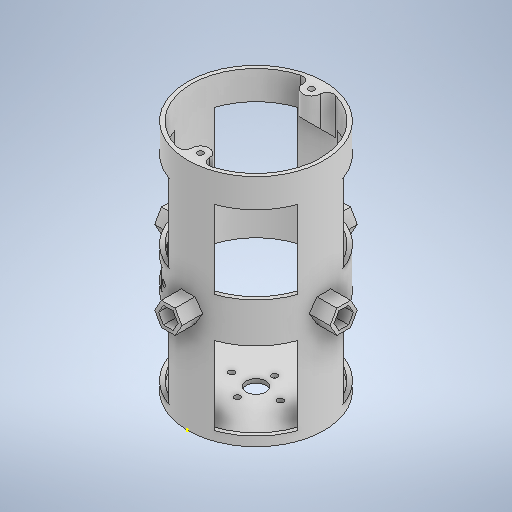
# Autodesk Inventor part: main_body
Saved by Autodesk Inventor 2025.3 (Build 293356000, 356)
## iProperties
Created: 2025-04-16
Part Number: main_body
Material: Generic
Document SubType Name: Modeling
Designer: Owner
Density: 1 g/cm^3
Appearance: Default
Author: Owner
Autodesk Inventor part; units mm, degrees
ref_plane "XZ Plane" through (0, 0, 0) normal (0, 1, 0) x (-1, 0, 0)
sketch "Sketch1" plane through (0, 0, 0) normal (0, 1, 0) x (-1, 0, 0)
  circle A0 centre (0, 0) radius 35
  dimension "d0" = 70
  constraints: 1 centre point, 1 coincident
  measures "d0" diameter of A0
extrude "Extrusion1" add sketch "Sketch1" along normal blind 120
shell "Shell1" thickness 2 removed faces 1 at (1.9985, 120, 11.019)
sketch "Sketch4" plane through (0, 120, 0) normal (0, 1, 0) x (1, 0, 0)
  circle A0 centre (0, 28.5) radius 4.5
  circle A1 centre (0, 0) radius 33 projected
  circle A2 centre (0, 28.5) radius 1.5
  line L0 (4.5, 28.5) -> (4.5, 32.6917)
  line L1 (0, 49) -> (0, -49) projected
  line L2 (-4.5, 28.5) -> (-4.5, 32.6917)
  point P0 (0, 33)
  dimension "d15" = 9
  dimension "d16" = 3
  constraints: 4 end point, 4 point on circle, 2 centre point, 2 tangent, 2 vertical, 1 coincident, 1 point on line
  measures "d15" diameter of A0
  measures "d16" diameter of A2
extrude "Extrusion2" add sketch "Sketch4" against normal blind 20 separate body contours A0 L1 A2 | A0 A1 L0 | L1 A2 A0 | A0 L2 A1
sketch "Sketch5" plane through (0, 0, 0) normal (1, 0, 0) x (0, 1, 0)
  line L0 (2, -33) -> (120, -33) projected
  line L1 (109, -24) -> (100, -33)
  line L2 (100, -24) -> (100, -28.5) projected
  line L3 (100, -33) -> (100, -24)
  line L4 (100, -24) -> (109, -24)
  point P0 (0, 0)
  point P1 (105.4104, -33)
  point P2 (130, -33)
  dimension "d60" = 45
  constraints: 6 end point, 3 point on line, 1 perpendicular, 1 vertical
  measures "d60" angle of L3 L1
extrude "Extrusion3" cut sketch "Sketch5" along normal mid plane 10 bodies 2
mirror "Mirror2" about plane through (0, 0, 0) normal (0, 0, 1) of "Extrusion3", "Extrusion2" bodies 2
combine bodies "Combine2" operation type add bodies to combine 2 1
sketch "Sketch6" plane through (0, 0, 0) normal (0, -1, 0) x (1, 0, 0)
  circle A0 centre (0, 9.5) radius 1.55
  circle A1 centre (0, -9.5) radius 1.55
  circle A2 centre (-12.5, 0) radius 1.55
  circle A3 centre (12.5, 0) radius 1.55
  circle A4 centre (0, 0) radius 20
  line L0 (0, 0) -> (14.1421, -14.1421)
  line L1 (0, -49) -> (0, 49) projected
  circle A5 centre (14.1421, -14.1421) radius 5
  circle A6 centre (0, 0) radius 5
  dimension "d69" = 40
  dimension "d35" = 3.1
  dimension "d36" = 3.1
  dimension "d37" = 3.1
  dimension "d38" = 3.1
  dimension "d39" = 19
  dimension "d40" = 25
  dimension "d41" = 9.5
  dimension "d42" = 12.5
  dimension "d71" = 45
  dimension "d72" = 10
  dimension "d73" = 10
  constraints: 6 centre point, 3 coincident, 2 end point, 3 other
  measures "d35" diameter of A0
  measures "d36" diameter of A1
  measures "d37" diameter of A2
  measures "d38" diameter of A3
  measures "d39" distance of A0.centre A1.centre
  measures "d40" distance of A2.centre A3.centre
  measures "d41" distance of point (0, 0) A0.centre
  measures "d42" distance of A3.centre point (0, 0)
  measures "d71" angle of L1 L0
  measures "d72" diameter of A5
  measures "d73" diameter of A6
extrude "Extrusion4" cut sketch "Sketch6" against normal through all contours A0 L1 | L1 A0 | A6 L0 L1 | L1 A6 | L0 A6 L1 | A5 A4 | A4 L0 A5 | A5 L0 A4 | L1 A1 | A1 L1 | A2 | A3 bodies 2
ref_plane "Work Plane1" through (0, 0, 35) normal (0, 0, 1) x (1, 0, 0)
sketch "Sketch7" plane through (0, 0, 35) normal (0, 0, 1) x (1, 0, 0)
  point P0 (0, 0)
sketch "Sketch8" plane through (0, 0, 35) normal (0, 0, 1) x (1, 0, 0)
  line L0 (2.5, 59.3301) -> (5, 55)
  line L1 (5, 55) -> (2.5, 50.6699)
  line L2 (2.5, 50.6699) -> (-2.5, 50.6699)
  line L3 (-2.5, 50.6699) -> (-5, 55)
  line L4 (-5, 55) -> (-2.5, 59.3301)
  line L5 (-2.5, 59.3301) -> (2.5, 59.3301)
  line L6 (35, 0) -> (-35, 0) projected
  line L7 (7, 55) -> (3.5, 48.9378)
  line L8 (3.5, 48.9378) -> (-3.5, 48.9378)
  line L9 (-3.5, 48.9378) -> (-7, 55)
  line L10 (-7, 55) -> (-3.5, 61.0622)
  line L11 (-3.5, 61.0622) -> (3.5, 61.0622)
  line L12 (3.5, 61.0622) -> (7, 55)
  point P0 (0, 0)
  point P1 (0, 55)
  point P2 (0, 55)
  point P3 (0, 48.9378)
  point P4 (0, 61.0622)
  dimension "d46" = 55
  dimension "d65" = 10
  dimension "d66" = 14
  constraints: 24 end point, 2 midpoint, 2 parallel, 1 coincident, 26 other
  measures "d46" distance from line of L6 point (0, 55)
  measures "d65" distance of L3.end L0.end
  measures "d66" distance of L9.end L7.start
extrude "Extrusion5" add sketch "Sketch8" against normal up to surface round surface about axis through (0, 0, 0) along (0, 1, 0) radius 35 far side no bodies 2
ref_plane "Work Plane2" through (0, 0, 0) normal (-0.7071068, 0, 0.7071068) x (0, -1, 0)
ref_plane "Work Plane3" through (-24.7487, 0, 24.7487) normal (-0.7071068, 0, 0.7071068) x (0, -1, 0)
sketch "Sketch10" plane through (-24.7487, 0, 24.7487) normal (-0.7071068, 0, 0.7071068) x (0, -1, 0)
  line L0 (-49.5, 7.75) -> (-60.5, 7.75)
  line L1 (-60.5, 7.75) -> (-60.5, -7.75)
  line L2 (-60.5, -7.75) -> (-49.5, -7.75)
  line L3 (-49.5, -7.75) -> (-49.5, 7.75)
  line L4 (-49.5, 7.75) -> (-60.5, -7.75) construction
  line L5 (-60.5, 7.75) -> (-49.5, -7.75) construction
  circle A0 centre (-55, -10.25) radius 2.5
  circle A1 centre (-55, -10.25) radius 1.5
  line L6 (12.1, 0) -> (-72.6, 0) projected
  circle A2 centre (-55, 10.25) radius 2.5
  circle A3 centre (-55, 10.25) radius 1.5
  line L7 (0, 35) -> (0, -35) projected
  point P0 (0, 0)
  point P1 (-55, 0)
  dimension "d54" = 11
  dimension "d55" = 15.5
  dimension "d56" = 5
  dimension "d57" = 3
  dimension "d67" = 55
  dimension "d68" = 55
  constraints: 12 end point, 4 centre point, 2 coincident, 2 midpoint, 2 parallel, 2 symmetric about line, 1 horizontal, 1 perpendicular, 1 point on line, 1 tangent, 2 other
  measures "d54" distance of L2.end L1.end
  measures "d55" distance of L1.end L0.end
  measures "d56" diameter of A0
  measures "d57" diameter of A1
  measures "d67" distance of point (0, 0) point (-55, 0)
  measures "d68" distance from line of L7 A0.centre
extrude "Extrusion7" cut sketch "Sketch10" against normal up to surface contours L3 L6 L1 L0 | L3 L2 L1 L6 | A1 | A3 round surface about axis through (0, 0, 0) along (0, 1, 0) radius 33 far side no bodies 2
fillet "Face Fillet13" radius 3.42 1 edges at (4.5, 110.1541, -32.6917)
fillet "Face Fillet14" radius 3.42 1 edges at (4.5, 110.1541, 32.6917)
fillet "Face Fillet15" radius 3.42 1 edges at (-4.5, 110.1541, -32.6917)
fillet "Face Fillet16" radius 3.42 1 edges at (-4.5, 110.1541, 32.6917)
sketch "Sketch13" plane through (-24.7487, 0, 24.7487) normal (-0.7071068, 0, 0.7071068) x (0, -1, 0)
  line L0 (-65.25, -15) -> (-105.25, -15)
  line L1 (-105.25, -15) -> (-105.25, 15)
  line L2 (-105.25, 15) -> (-65.25, 15)
  line L3 (-65.25, 15) -> (-65.25, -15)
  line L4 (-65.25, -15) -> (-105.25, 15) construction
  line L5 (-105.25, -15) -> (-65.25, 15) construction
  line L6 (-60.5, 7.75) -> (-60.5, -7.75) projected
  line L7 (-4.75, -15) -> (-44.75, -15)
  line L8 (-44.75, -15) -> (-44.75, 15)
  line L9 (-44.75, 15) -> (-4.75, 15)
  line L10 (-4.75, 15) -> (-4.75, -15)
  line L11 (-4.75, -15) -> (-44.75, 15) construction
  line L12 (-44.75, -15) -> (-4.75, 15) construction
  line L13 (-49.5, -7.75) -> (-49.5, 7.75) projected
  ellipse E0 centre (-104.5, 25.7528) end of major axis (-101.3403, 28.9125) minor radius 1.8509 (-104.5, 23.3345) -> (-101.2049, 28.7303) ccw projected
  ellipse E1 centre (-104.5, 20.1525) end of major axis (-108.6575, 15.9951) minor radius 2.4354 (-104.5, 23.3345) -> (-104.5, 16.9706) ccw projected
  ellipse E2 centre (-104.5, 14.5523) end of major axis (-101.3403, 17.7119) minor radius 1.8509 (-101.2049, 16.2348) -> (-104.5, 16.9706) ccw projected
  line L14 (21.05, 0) -> (-126.3, 0) projected
  point P0 (0, 0)
  point P1 (-85.25, 0)
  point P2 (-24.75, 0)
  dimension "d78" = 40
  dimension "d79" = 30
  dimension "d80" = 4.75
  dimension "d81" = 40
  dimension "d82" = 30
  dimension "d83" = 4.75
  constraints: 24 end point, 4 midpoint, 4 parallel, 2 horizontal, 2 perpendicular, 2 point on line, 3 other
  measures "d78" distance of L1.end L2.end
  measures "d79" distance of L0.end L1.end
  measures "d80" distance between parallel lines of L6 L3
  measures "d81" distance of L8.end L9.end
  measures "d82" distance of L7.end L8.end
  measures "d83" distance between parallel lines of L13 L8
extrude "Extrusion10" cut sketch "Sketch13" against normal up to surface round surface about axis through (0, 0, 0) along (0, 1, 0) radius 33 far side no bodies 2
sketch "Sketch12" plane through (0, 0, 35) normal (0, 0, 1) x (1, 0, 0)
  line L0 (0, 59.3301) -> (-2.5, 59.3301) projected
  line L1 (-2.5, 59.3301) -> (-5, 55) projected
  line L2 (-5, 55) -> (-2.5, 50.6699) projected
  line L3 (-2.5, 50.6699) -> (0, 50.6699) projected
  line L4 (0, 50.6699) -> (2.5, 50.6699) projected
  line L5 (2.5, 50.6699) -> (5, 55) projected
  line L6 (5, 55) -> (2.5, 59.3301) projected
  line L7 (2.5, 59.3301) -> (0, 59.3301) projected
  line L8 (0, 50.6699) -> (-2.5, 50.6699) projected
  line L9 (-2.5, 50.6699) -> (-5, 55) projected
  line L10 (-5, 55) -> (-2.5, 59.3301) projected
  line L11 (-2.5, 59.3301) -> (0, 59.3301) projected
  line L12 (0, 59.3301) -> (2.5, 59.3301) projected
  line L13 (2.5, 59.3301) -> (5, 55) projected
  line L14 (5, 55) -> (2.5, 50.6699) projected
  line L15 (2.5, 50.6699) -> (0, 50.6699) projected
  line L16 (0, 48.9378) -> (3.5, 48.9378) projected
  line L17 (3.5, 48.9378) -> (7, 55) projected
  line L18 (7, 55) -> (3.5, 61.0622) projected
  line L19 (3.5, 61.0622) -> (0, 61.0622) projected
  line L20 (0, 61.0622) -> (-3.5, 61.0622) projected
  line L21 (-3.5, 61.0622) -> (-7, 55) projected
  line L22 (-7, 55) -> (-3.5, 48.9378) projected
  line L23 (-3.5, 48.9378) -> (0, 48.9378) projected
  point P0 (0, 0)
extrude "Extrusion9" add sketch "Sketch12" along normal blind 10 bodies 2
mirror "Mirror5" about plane through (0, 0, 0) normal (0, 0, 1) of "Extrusion9", "Extrusion5" bodies 2
mirror "Mirror6" about plane through (0, 0, 0) normal (-0.7071068, 0, 0.7071068) of "Extrusion9", "Extrusion5", "Mirror5" bodies 2
mirror "Mirror7" about plane through (0, 0, 0) normal (-0.7071068, 0, 0.7071068) of "Extrusion10" bodies 2
mirror "Mirror8" about plane through (0, 0, 0) normal (0, 0, 1) of "Extrusion10", "Mirror7" bodies 2
body "Solid2"
